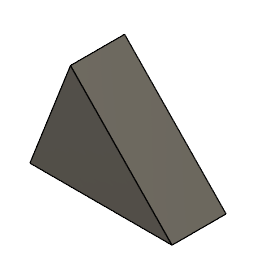
replay (Autodesk Fusion 360 design; units mm, degrees)
Autodesk Fusion 360 part; units mm, degrees
sketch "草图1" plane through (0, 0, 0) normal (0, 0, 1) x (1, 0, 0)
  line L0 (54, -8) -> (24, 23)
  line L1 (24, 23) -> (12, -8)
  line L2 (12, -8) -> (54, -8)
extrude "拉伸1" add sketch "草图1" along normal blind 16
